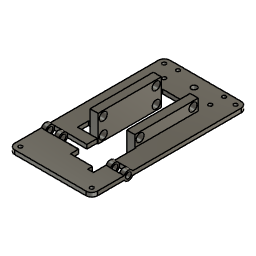
oke v4 (Autodesk Fusion 360 design; units mm, degrees)
Autodesk Fusion 360 part; units mm, degrees
note: some values were not read from the file. Set by a fixed rule: which sketch regions a step uses.
sketch "Sketch1" plane through (0, 0, 0) normal (0, 0, 1) x (1, 0, 0)
  line L0 (-27.6756, 45.9596) -> (34.3244, 45.9596)
  line L1 (-32.6756, 40.9596) -> (-32.6756, -84.0404)
  line L2 (-27.6756, -89.0404) -> (34.3244, -89.0404)
  line L3 (39.3244, -84.0404) -> (39.3244, 40.9596)
  arc A0 (39.3244, 40.9596) -> (34.3244, 45.9596) centre (34.3244, 40.9596) ccw
  arc A1 (-27.6756, 45.9596) -> (-32.6756, 40.9596) centre (-27.6756, 40.9596) ccw
  arc A2 (-32.6756, -84.0404) -> (-27.6756, -89.0404) centre (-27.6756, -84.0404) ccw
  arc A3 (34.3244, -89.0404) -> (39.3244, -84.0404) centre (34.3244, -84.0404) ccw
  circle A4 centre (-27.6756, 40.9596) radius 1.6
  circle A5 centre (34.3244, 40.9596) radius 1.6
  circle A6 centre (34.3244, -84.0404) radius 1.6
  circle A7 centre (-27.6756, -84.0404) radius 1.6
  circle A8 centre (3.3244, 35.9596) radius 2.5
  circle A9 centre (-16.6756, 41.9596) radius 1.6
  circle A10 centre (-16.6756, 29.9596) radius 1.6
  circle A11 centre (23.3244, 41.9596) radius 1.6
  circle A12 centre (23.3244, 29.9596) radius 1.6
  line L4 (-9.1756, 20.9596) -> (-9.1756, -35.0404)
  line L5 (-9.1756, 20.9596) -> (15.8244, 20.9596)
  line L6 (15.8244, 20.9596) -> (15.8244, -35.0404)
  line L7 (-9.1756, -35.0404) -> (15.8244, -35.0404)
  line L8 (-17.4618, -35.0396) -> (-17.4618, -71.7396)
  line L9 (-17.4618, -71.7396) -> (23.5382, -71.7396)
  line L10 (23.5382, -71.7396) -> (23.5382, -35.0396)
  line L11 (-17.4618, -35.0396) -> (23.5382, -35.0396)
  line L12 (-28.8687, -53.3412) -> (-21.2687, -53.3412)
  line L13 (-28.8687, -53.3412) -> (-28.8687, -60.9412)
  line L14 (-21.2687, -53.3412) -> (-21.2687, -60.9412)
  line L15 (-28.8687, -60.9412) -> (-21.2687, -60.9412)
  line L16 (-60, -39) -> (-60, -28)
  line L17 (-17.4618, -71.7396) -> (-17.4618, -60.7396)
  line L18 (-17.4618, -60.7396) -> (-0.4618, -60.7396)
  line L19 (-17.4618, -71.7396) -> (-0.4618, -71.7396)
  line L20 (-17.4618, -53.3896) -> (-0.4625, -53.5429)
  line L21 (-0.4625, -53.5429) -> (-0.3813, -44.5432)
  line L22 (-0.3813, -44.5432) -> (-17.4618, -44.5432)
  line L23 (-17.4618, -44.5432) -> (-17.4618, -53.3896)
  line L24 (18.5382, -71.7396) -> (18.5382, -67.7396)
  line L25 (18.5382, -67.7396) -> (0.5382, -67.7396)
  line L26 (0.5382, -71.7396) -> (18.5382, -71.7396)
  line L27 (0.5382, -67.7396) -> (-0.4618, -67.7396)
  line L28 (-0.4618, -60.7396) -> (-0.4618, -67.7396)
  line L29 (27.6313, -53.3412) -> (35.2313, -53.3412)
  line L30 (35.2313, -53.3412) -> (35.2313, -60.9412)
  line L31 (27.6313, -53.3412) -> (27.6313, -60.9412)
  line L32 (27.6313, -60.9412) -> (35.2313, -60.9412)
  point P0 (-32.6756, 45.9596)
  point P1 (39.3244, 45.9596)
  point P2 (-32.6756, -89.0404)
  point P3 (39.3244, -89.0404)
  point P4 (39.3244, 20.9596)
  dimension "d1" = 72
  dimension "d2" = 135
  dimension "d3" = 72
  dimension "d4" = 110
  dimension "d5" = 5
  dimension "d6" = 5
  dimension "d7" = 5
  dimension "d8" = 5
  dimension "d9" = 3.2
  dimension "d10" = 3.2
  dimension "d11" = 3.2
  dimension "d12" = 3.2
  dimension "d14" = 5
  dimension "d19" = 10
  dimension "d23" = 3.2
  dimension "d24" = 3.2
  dimension "d25" = 3.2
  dimension "d26" = 3.2
  dimension "d27" = 56
  dimension "d28" = 25
  dimension "d29" = 56
  dimension "d32" = 36.7
  dimension "d33" = 41
  dimension "d34" = 36.7
  dimension "d35" = 7.6
  dimension "d37" = 7.6
  dimension "d38" = 7.6
  dimension "d39" = 11
  dimension "d42" = 17
  dimension "d43" = 9
  dimension "d46" = 4
  dimension "d48" = 7.6
  dimension "d49" = 7.6
  dimension "d50" = 7.6
  constraint horizontal L0
  constraint perpendicular L0 L1
  constraint perpendicular L1 L2
  constraint perpendicular L0 L3
  constraint coincident P1 L0
  constraint coincident P4 L3
  constraint tangent L0 A0
  constraint tangent L3 A0
  constraint coincident P0 L1
  constraint coincident P0 L0
  constraint tangent L1 A1
  constraint tangent L0 A1
  constraint coincident P2 L1
  constraint coincident P2 L2
  constraint tangent L1 A2
  constraint tangent L2 A2
  constraint coincident P3 L2
  constraint coincident P3 L3
  constraint tangent L2 A3
  constraint tangent L3 A3
  constraint concentric A1 A4
  constraint concentric A0 A5
  constraint concentric A3 A6
  constraint concentric A2 A7
  constraint parallel L1 L4
  constraint perpendicular L4 L5
  constraint perpendicular L5 L6
  constraint vertical L8
  constraint perpendicular L1 L9
  constraint perpendicular L9 L10
  constraint perpendicular L1 L12
  constraint perpendicular L12 L13
  constraint perpendicular L12 L14
  constraint vertical L16
  constraint perpendicular L9 L17
  constraint perpendicular L17 L18
  constraint coincident L9 L19.end
  constraint midpoint L8 L20.start
  constraint perpendicular L20 L21
  constraint coincident L8 L22.end
  constraint perpendicular L8 L22
  constraint coincident L9 L24.start
  constraint perpendicular L24 L25
  constraint coincident L9 L26.start
  constraint perpendicular L24 L26
  constraint perpendicular L27 L28
  constraint perpendicular L29 L30
  constraint perpendicular L29 L31
  measures "d1" distance of P0 P1
  measures "d2" distance of P0 P2
  measures "d3" distance of P2 P3
  measures "d4" distance of P3 P4
  measures "d5" radius of A0
  measures "d6" radius of A1
  measures "d7" radius of A2
  measures "d8" radius of A3
  measures "d9" diameter of A4
  measures "d10" diameter of A5
  measures "d11" diameter of A6
  measures "d12" diameter of A7
  measures "d14" diameter of A8
  measures "d19" distance of L0 A8.centre
  measures "d23" diameter of A9
  measures "d24" diameter of A10
  measures "d25" diameter of A11
  measures "d26" diameter of A12
  measures "d27" distance of L4.start L4.end
  measures "d28" distance of L4.start L5.end
  measures "d29" distance of L5.end L6.end
  measures "d32" distance of L8.start L8.end
  measures "d33" distance of L8.end L9.end
  measures "d34" distance of L9.end L10.end
  measures "d35" distance of L12.start L12.end
  measures "d37" distance of L12.start L13.end
  measures "d38" distance of L12.end L14.end
  measures "d39" distance of L8.end L17.end
  measures "d42" distance of L20.start L20.end
  measures "d43" distance of L20.end L21.end
  measures "d46" distance of L24.start L24.end
  measures "d48" distance of L29.start L29.end
  measures "d49" distance of L29.end L30.end
  measures "d50" distance of L29.start L31.end
extrude "Extrude1" add sketch "Sketch1" along normal blind 3.5 contours L0 L1 L2 L3 A0 A1 A2 A3 | L8 L20 L21 L22 L23 | L8 L9 L17 L18 L19 L24 L25 L26 L27 L28 makes body 1
sketch "Sketch2" plane through (0, 0, 0) normal (1, 0, 0) x (0, 1, 0)
  circle A0 centre (-58.9237, 12.2782) radius 4
  circle A1 centre (-58.9237, 12.2782) radius 2.5
  dimension "d53" = 8
  dimension "d54" = 5
  constraint concentric A0 A1
  measures "d53" diameter of A0
  measures "d54" diameter of A1
extrude "Extrude3" add sketch "Sketch2" along normal blind 72 separate body makes body 2
move_body "Align1" bodies 2 to x (0, -1, 0) y (1, 0, 0) z (0, 0, 1) at (26.2481, -58.9237, -8.7782)
move_body "Align2" bodies 2 to x (1, 0, 0) y (0, 1, 0) z (0, 0, 1) at (72, 0, 0)
move_body "Move3" bodies 2 to x (0, 1, 0) y (-1, 0, 0) z (0, 0, 1) at (-94.8493, -166.9981, 0)
move_body "Move4" bodies 2 to x (1, 0, 0) y (0, 1, 0) z (0, 0, 1) at (3.25, 70.5, 0)
move_body "Move5" bodies 2 to x (1, 0, 0) y (0, 1, 0) z (0, 0, 1) at (0, 0, -1.7)
combine "Combine1" operation add target body 1 tool bodies 2
sketch "Sketch3" plane through (0, 0, 0) normal (1, 0, 0) x (0, 1, 0)
  circle A0 centre (-60, 35) radius 2.5
  dimension "d59" = 5
  measures "d59" diameter of A0
extrude "Extrude4" add sketch "Sketch3" along normal blind 300 separate body makes body 3
move_body "Move6" bodies 3 to x (1, 0, 0) y (0, 1, 0) z (0, 0, 1) at (0, 2.5942, -33.2053)
move_body "Move7" bodies 3 to x (1, 0, 0) y (0, 1, 0) z (0, 0, 1) at (0, 0.23, 0)
move_body "Move8" bodies 3 to x (1, 0, 0) y (0, 1, 0) z (0, 0, 1) at (-60, 0, 0)
combine "Combine2" operation cut target body 1 tool bodies 3
extrude "Extrude5" add sketch "Sketch1" along normal blind 500 separate body contours L12 L13 L14 L15 makes body 4
move_body "Move9" bodies 4 to x (1, 0, 0) y (0, 1, 0) z (0, 0, 1) at (0, 0, -22)
combine "Combine3" operation cut target body 1 tool bodies 4
extrude "Extrude6" add sketch "Sketch1" along normal blind 500 separate body contours L29 L30 L31 L32 makes body 5
move_body "Move10" bodies 5 to x (1, 0, 0) y (0, 1, 0) z (0, 0, 1) at (0, 0, -14)
combine "Combine4" operation cut target body 1 tool bodies 5
extrude "Extrude7" cut sketch "Sketch1" along normal blind 30 contours L7 L8 L9 L10 L11 L18 L20 L21 L22 L24 L25 L27 L28 bodies 1
extrude "Extrude8" cut sketch "Sketch1" against normal blind 7 contours L7 L8 L9 L10 L11 L18 L20 L21 L22 L24 L25 L27 L28 bodies 1
sketch "Sketch6" plane through (0, 0, 0) normal (1, 0, 0) x (0, 1, 0)
  circle A0 centre (2.5, 8.5) radius 4
  circle A1 centre (2.5, 8.5) radius 2.5
  dimension "d70" = 8
  dimension "d71" = 5
  constraint concentric A0 A1
  measures "d70" diameter of A0
  measures "d71" diameter of A1
extrude "Extrude9" add sketch "Sketch6" along normal blind 74 separate body makes body 6
sketch "Sketch7" plane through (0, 0, 3.5) normal (0, 0, 1) x (-1, 0, 0)
  line L0 (-23.5382, 53.5529) -> (-27.6313, 53.5529)
  line L1 (-27.6313, 53.5529) -> (-27.6313, 53.3412)
  line L2 (-27.6313, 53.3412) -> (-35.2313, 53.3412)
  line L3 (-35.2313, 53.3412) -> (-35.2313, 53.5529)
  line L4 (-35.2313, 53.5529) -> (-39.3244, 53.5529)
  line L5 (-39.3244, 53.5529) -> (-39.3244, -40.9596)
  arc A0 (-39.3244, -40.9596) -> (-34.3244, -45.9596) centre (-34.3244, -40.9596) ccw
  line L6 (-34.3244, -45.9596) -> (27.6756, -45.9596)
  arc A1 (27.6756, -45.9596) -> (32.6756, -40.9596) centre (27.6756, -40.9596) ccw
  line L7 (32.6756, -40.9596) -> (32.6756, 53.5529)
  line L8 (32.6756, 53.5529) -> (28.8687, 53.5529)
  line L9 (28.8687, 53.5529) -> (28.8687, 53.3412)
  line L10 (28.8687, 53.3412) -> (21.2687, 53.3412)
  line L11 (21.2687, 53.3412) -> (21.2687, 53.5529)
  line L12 (21.2687, 53.5529) -> (17.4618, 53.5529)
  line L13 (17.4618, 53.5529) -> (17.4618, 53.3896)
  line L14 (17.4618, 53.3896) -> (0.4625, 53.5429)
  line L15 (0.4625, 53.5429) -> (0.3813, 44.5432)
  line L16 (0.3813, 44.5432) -> (17.4618, 44.5432)
  line L17 (17.4618, 44.5432) -> (17.4618, 35.0396)
  line L18 (17.4618, 35.0396) -> (9.1756, 35.0396)
  line L19 (9.1756, 35.0396) -> (9.1756, -20.9596)
  line L20 (9.1756, -20.9596) -> (-15.8244, -20.9596)
  line L21 (-15.8244, -20.9596) -> (-15.8244, 35.0396)
  line L22 (-15.8244, 35.0396) -> (-23.5382, 35.0396)
  line L23 (-23.5382, 35.0396) -> (-23.5382, 53.5529)
  circle A2 centre (-23.3244, -29.9596) radius 1.6
  circle A3 centre (16.6756, -29.9596) radius 1.6
  circle A4 centre (-34.3244, -40.9596) radius 1.6
  circle A5 centre (16.6756, -41.9596) radius 1.6
  circle A6 centre (-3.3244, -35.9596) radius 2.5
  circle A7 centre (-23.3244, -41.9596) radius 1.6
  circle A8 centre (27.6756, -40.9596) radius 1.6
  line L24 (-15.8244, 35.0397) -> (-22.8244, 35.0397)
  line L25 (-22.8244, 35.0397) -> (-22.8244, -19.9603)
  line L26 (-22.8244, -19.9603) -> (-15.8244, -19.9603)
  line L27 (-15.8244, -19.9603) -> (-15.8244, 35.0397)
  dimension "d74" = 7
  dimension "d75" = 55
  constraint coincident L21 L24.start
  constraint perpendicular L21 L24
  constraint perpendicular L24 L25
  constraint coincident L21 L26.end
  constraint perpendicular L21 L26
  measures "d74" distance of L24.start L24.end
  measures "d75" distance of L24.end L25.end
sketch "Sketch9" plane through (0, 0, 3.5) normal (0, 0, 1) x (1, 0, 0)
  line L0 (-9.1755, -35.0462) -> (-16.1755, -35.0462)
  line L1 (-16.1755, -35.0462) -> (-16.1755, 19.9538)
  line L2 (-16.1755, 19.9538) -> (-9.1755, 19.9538)
  line L3 (-9.1755, 19.9538) -> (-9.1755, -35.0462)
  dimension "d81" = 7
  dimension "d82" = 55
  dimension "d83" = 7
  constraint horizontal L0
  constraint perpendicular L0 L1
  constraint perpendicular L1 L2
  measures "d81" distance of L0.start L0.end
  measures "d82" distance of L0.end L1.end
  measures "d83" distance of L1.end L2.end
extrude "Extrude11" add sketch "Sketch9" sketch "Sketch7" along normal blind 9.75 of sketch 2 contours L21 L22 L24 L25 L26 L27 bodies 1
extrude "Extrude12" add sketch "Sketch9" sketch "Sketch7" against normal blind 13.25 of sketch 2 contours L21 L22 L24 L25 L26 L27 bodies 1
sketch "Sketch11" plane through (22.8244, 0, 0) normal (1, 0, 0) x (0, 1, 0)
  line L0 (-35.0396, 3.5) -> (19.9603, 3.5)
  line L1 (19.9603, 3.5) -> (19.9603, 13.25)
  line L2 (19.9603, 13.25) -> (-35.0396, 13.25)
  line L3 (-35.0396, 13.25) -> (-35.0396, 3.5)
  line L4 (-35.0396, 13.25) -> (-35.0284, 13.25) construction
  circle A0 centre (-30.5396, 8.75) radius 3.5
  line L5 (-35.0396, 8.75) -> (-30.5396, 8.75)
  line L6 (-30.5396, 8.75) -> (-30.5396, 13.25)
  line L7 (19.9603, 8.75) -> (15.4603, 8.75)
  line L8 (15.4603, 8.75) -> (15.4603, 13.25)
  circle A1 centre (15.4603, 8.75) radius 3.5
  dimension "d91" = 7
  dimension "d94" = 4.5
  dimension "d95" = 4.5
  dimension "d96" = 4.5
  dimension "d97" = 4.5
  dimension "d98" = 7
  constraint horizontal L4
  constraint coincident L2.end L3.start
  constraint coincident L3 L5.start
  constraint perpendicular L3 L5
  constraint coincident L2 L6.end
  constraint perpendicular L2 L6
  constraint coincident A0.centre L5.end
  constraint coincident L1 L7.start
  constraint perpendicular L1 L7
  constraint perpendicular L7 L8
  constraint coincident L2 L8.end
  constraint coincident L7.end L8.start
  measures "d91" diameter of A0
  measures "d94" distance of L5.start A0.centre
  measures "d95" distance of A0.centre L6.end
  measures "d96" distance of L7.start L7.end
  measures "d97" distance of L7.end L8.end
  measures "d98" diameter of A1
extrude "Extrude13" cut sketch "Sketch11" against normal blind 82 contours A0 L5 L6 | A0 L5 L6 | L7 L8 A1 | L7 L8 A1 bodies 1
sketch "Sketch12" plane through (22.8244, 0, 0) normal (1, 0, 0) x (0, 1, 0)
  line L0 (19.9603, 0) -> (-35.0396, 0)
  line L1 (-35.0396, 0) -> (-35.0396, -9.75)
  line L2 (-35.0396, -9.75) -> (19.9603, -9.75)
  line L3 (19.9603, -9.75) -> (19.9603, 0)
  line L4 (-35.0396, -5.25) -> (-30.5396, -5.25)
  line L5 (-30.5396, -5.25) -> (-30.5396, -9.75)
  circle A0 centre (-30.5396, -5.25) radius 3.5
  line L6 (15.5072, -9.75) -> (15.5072, -5.25)
  line L7 (15.5072, -5.25) -> (20.0072, -5.25)
  circle A1 centre (15.5072, -5.25) radius 3.5
  dimension "d101" = 4.5
  dimension "d102" = 4.5
  dimension "d103" = 7
  dimension "d104" = 4.5
  dimension "d105" = 4.5
  dimension "d106" = 7
  constraint coincident L1 L4.start
  constraint perpendicular L1 L4
  constraint perpendicular L2 L5
  constraint coincident L2 L5.end
  constraint coincident L4.end L5.start
  constraint coincident L2 L6.start
  constraint perpendicular L2 L6
  constraint perpendicular L3 L7
  constraint coincident L6.end L7.start
  measures "d101" distance of L4.start L4.end
  measures "d102" distance of L4.end L5.end
  measures "d103" diameter of A0
  measures "d104" distance of L6.start L6.end
  measures "d105" distance of L6.end L7.end
  measures "d106" diameter of A1
extrude "Extrude14" cut sketch "Sketch12" against normal blind 1000 contours L6 L7 A1 | L6 L7 A1 | L4 L5 A0 | L4 L5 A0 bodies 1
extrude "Extrude10" [suppressed]
fillet "Fillet1" [suppressed]
hidden bodies 6
